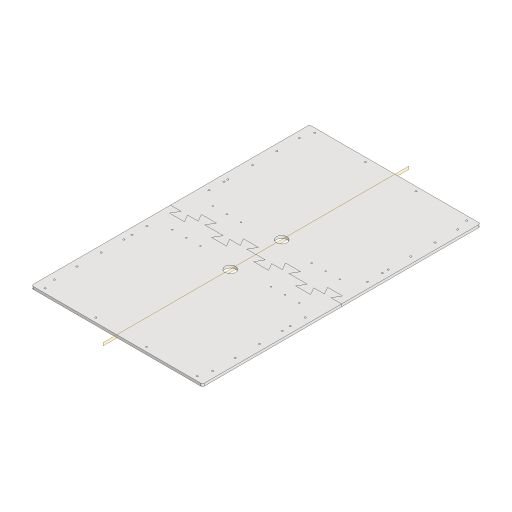
# Autodesk Inventor part: platform
Saved by Autodesk Inventor 2023.2 (Build 272271030, 271C)
## iProperties
Created: 2024-10-30
Part Number: platform
Material: Типовые
Document SubType Name: Modeling
Designer: I9232
Density: 1 g/cm^3
Appearance: По умолчанию
Author: I9232
Autodesk Inventor part; units mm, degrees
ref_plane "XZ Plane" through (0, 0, 0) normal (0, 1, 0) x (-1, 0, 0)
ref_plane "XY Plane" through (0, 0, 0) normal (0, 0, 1) x (1, 0, 0)
sketch "Эскиз1" plane through (0, 0, 0) normal (0, 1, 0) x (-1, 0, 0)
  line L0 (200, 325) -> (-200, 325)
  line L1 (-200, 325) -> (-200, -325)
  line L2 (-200, -325) -> (200, -325)
  line L3 (200, -325) -> (200, 325)
  line L4 (200, 325) -> (-200, -325) construction
  line L5 (-200, 325) -> (200, -325) construction
  point P0 (0, 0)
  dimension "d0" = 650
  dimension "d1" = 400
  constraints: 12 end point, 2 midpoint, 2 parallel, 1 horizontal, 1 perpendicular
  measures "d0" distance of L0.end L1.end
  measures "d1" distance of L1.end L2.end
extrude "Выдавливание1" add sketch "Эскиз1" along normal mid plane 6
fillet "Сопряжение1" radius 4 4 edges at (-200, 0, -325) (200, 0, -325) (200, 0, 325) (-200, 0, 325)
sketch "Эскиз3" plane through (0, 3, 0) normal (0, 1, 0) x (1, 0, 0)
  circle A0 centre (185, -105) radius 2
  arc A1 (-200, -321) -> (-196, -325) centre (-196, -321) ccw projected
  line L0 (-196, -325) -> (196, -325) projected
  arc A2 (196, -325) -> (200, -321) centre (196, -321) ccw projected
  line L1 (200, -321) -> (200, 321) projected
  arc A3 (200, 321) -> (196, 325) centre (196, 321) ccw projected
  line L2 (196, 325) -> (-196, 325) projected
  arc A4 (-196, 325) -> (-200, 321) centre (-196, 321) ccw projected
  line L3 (-200, 321) -> (-200, -321) projected
  line L4 (185, -413) -> (185, 413) construction
  circle A5 centre (-178, 315) radius 2
  line L5 (280, 0) -> (-280, 0) construction
  line L6 (-200, 315) -> (-183.7984, 315) construction
  circle A6 centre (-59.5, 315) radius 2
  circle A7 centre (59, 315) radius 2
  circle A8 centre (177.5, 315) radius 2
  circle A9 centre (185, -286.5) radius 2
  circle A10 centre (185, -233.5) radius 2
  circle A11 centre (185, -177) radius 2
  circle A12 centre (185, -124) radius 2
  circle A13 centre (-178, -315) radius 2
  circle A14 centre (-59.5, -315) radius 2
  circle A15 centre (59, -315) radius 2
  circle A16 centre (177.5, -315) radius 2
  line L7 (0, -50) -> (0, 50) construction
  circle A17 centre (-185, -105) radius 2
  circle A18 centre (-185, -286.5) radius 2
  circle A19 centre (-185, -233.5) radius 2
  circle A20 centre (-185, -177) radius 2
  circle A21 centre (185, 286.5) radius 2
  circle A22 centre (185, 233.5) radius 2
  circle A23 centre (185, 177) radius 2
  circle A24 centre (185, 124) radius 2
  circle A25 centre (-185, 286.5) radius 2
  circle A26 centre (-185, 233.5) radius 2
  circle A27 centre (-185, 177) radius 2
  circle A28 centre (-185, 119) radius 2
  circle A29 centre (185, -70) radius 2
  circle A30 centre (185, 75) radius 2
  circle A31 centre (185, 110) radius 2
  circle A32 centre (-185, -105) radius 2
  circle A33 centre (-185, -70) radius 2
  circle A34 centre (-185, 75) radius 2
  circle A35 centre (-185, 110) radius 2
  circle A36 centre (-185, -124) radius 2
  point P0 (0, 0)
  point P1 (185, 325)
  point P2 (185, -103)
  point P3 (185, -107)
  point P4 (185, -325)
  point P5 (0, 0)
  dimension "d7" = 4
  dimension "d15" = 4
  dimension "d17" = 220
  dimension "d34" = 10
  dimension "d35" = 22
  dimension "d38" = 118.5
  dimension "d43" = 4
  dimension "d44" = 38.5
  dimension "d45" = 4
  dimension "d46" = 4
  dimension "d47" = 4
  dimension "d48" = 53
  dimension "d49" = 53
  dimension "d50" = 56.5
  dimension "d51" = 100
  dimension "d58" = 35
  dimension "d59" = 35
  dimension "d60" = 14
  constraints: 33 centre point, 20 symmetric about line, 6 end point, 3 equal radius, 3 horizontal, 2 midpoint, 2 point on line, 1 vertical, 40 other
  measures "d7" diameter of A0
  measures "d15" diameter of A5
  measures "d17" distance from line of L0 A0.centre
  measures "d34" distance between parallel lines of L2 L6
  measures "d35" distance of L6.start A5.centre
  measures "d38" distance of A5.centre A6.centre
  measures "d43" diameter of A9
  measures "d44" distance from line of L0 A9.centre
  measures "d45" diameter of A10
  measures "d46" diameter of A11
  measures "d47" diameter of A12
  measures "d48" distance of A10.centre A9.centre
  measures "d49" distance of A12.centre A11.centre
  measures "d50" distance of A11.centre A10.centre
  measures "d51" distance of L7.start L7.end
  measures "d58" distance of A29.centre A0.centre
  measures "d59" distance of A31.centre A30.centre
  measures "d60" distance of A24.centre A31.centre
extrude "Выдавливание3" cut sketch "Эскиз3" against normal up to surface (6 mm away) contours A0 | A5 | A6 | A7 | A8 | A9 | A10 | A11 | A12 | A13 | A14 | A15 | A16 | A17 | A18 | A19 | A20 | A21 | A22 | A23 | A24 | A25 | A26 | A27 | A28 | A29 | A30 | A31 | A33 | A34 | A35 | A36
sketch "Эскиз5" plane through (0, -3, 0) normal (0, -1, 0) x (1, 0, 0)
  circle A0 centre (148.4926, 47.4999) radius 1.5999 projected
  circle A1 centre (115.4927, 47.5002) radius 1.6002 projected
  circle A2 centre (82.4926, 47.4999) radius 1.5999 projected
  circle A3 centre (82.4928, -47.4999) radius 1.6002 projected
  circle A4 centre (115.4927, -47.5) radius 1.6001 projected
  circle A5 centre (148.4927, -47.5) radius 1.6001 projected
  circle A6 centre (-82.4927, 47.5) radius 1.5999 projected
  circle A7 centre (-115.4927, 47.5) radius 1.6 projected
  circle A8 centre (-148.4927, 47.4999) radius 1.5999 projected
  circle A9 centre (-148.4927, -47.5) radius 1.6 projected
  circle A10 centre (-115.4927, -47.5) radius 1.5999 projected
  circle A11 centre (-82.4926, -47.5) radius 1.6 projected
  point P0 (0, 0)
extrude "Выдавливание5" cut sketch "Эскиз5" against normal up to surface (6 mm away)
sketch "Эскиз6" plane through (0, -3, 0) normal (0, -1, 0) x (1, 0, 0)
  circle A0 centre (0, 60) radius 12.5
  circle A1 centre (0, -60) radius 12.5
  line L0 (0, 455) -> (0, -455) construction
  point P0 (0, 0)
  dimension "d61" = 25
  dimension "d62" = 25
  dimension "d63" = 60
  dimension "d64" = 60
  constraints: 2 centre point, 2 point on line
  measures "d61" diameter of A0
  measures "d62" diameter of A1
  measures "d63" distance of point (0, 0) A0.centre
  measures "d64" distance of point (0, 0) A1.centre
extrude "Выдавливание6" cut sketch "Эскиз6" against normal up to surface (6 mm away)
sketch "Эскиз7" plane through (0, -3, 0) normal (0, -1, 0) x (1, 0, 0)
  line L0 (200, 321) -> (200, -321) projected
  line L1 (200, 0) -> (175, 0)
  line L2 (175, 0) -> (185, -17.3205)
  line L3 (185, -17.3205) -> (150, -17.3205)
  line L4 (150, -17.3205) -> (160, 0)
  line L5 (160, 0) -> (135, 0)
  line L6 (-200, -321) -> (-200, 321) projected
  line L7 (135, 0) -> (145, 17.3205)
  line L8 (145, 17.3205) -> (110, 17.3205)
  line L9 (110, 17.3205) -> (120, 0)
  line L10 (-280, 0) -> (280, 0) construction
  line L11 (101.6669, 0) -> (76.6669, 0)
  line L12 (76.6669, 0) -> (86.6669, -17.3205)
  line L13 (86.6669, -17.3205) -> (51.6669, -17.3205)
  line L14 (51.6669, -17.3205) -> (61.6669, 0)
  line L15 (61.6669, 0) -> (36.6669, 0)
  line L16 (36.6669, 0) -> (46.6669, 17.3205)
  line L17 (46.6669, 17.3205) -> (11.6669, 17.3205)
  line L18 (11.6669, 17.3205) -> (21.6669, 0)
  line L19 (3.3338, 0) -> (-21.6662, 0)
  line L20 (-21.6662, 0) -> (-11.6662, -17.3205)
  line L21 (-11.6662, -17.3205) -> (-46.6662, -17.3205)
  line L22 (-46.6662, -17.3205) -> (-36.6662, 0)
  line L23 (-36.6662, 0) -> (-61.6662, 0)
  line L24 (-61.6662, 0) -> (-51.6662, 17.3205)
  line L25 (-51.6662, 17.3205) -> (-86.6662, 17.3205)
  line L26 (-86.6662, 17.3205) -> (-76.6662, 0)
  line L27 (-94.9993, 0) -> (-119.9993, 0)
  line L28 (-119.9993, 0) -> (-109.9993, -17.3205)
  line L29 (-109.9993, -17.3205) -> (-144.9993, -17.3205)
  line L30 (-144.9993, -17.3205) -> (-134.9993, 0)
  line L31 (-134.9993, 0) -> (-159.9993, 0)
  line L32 (-159.9993, 0) -> (-149.9993, 17.3205)
  line L33 (-149.9993, 17.3205) -> (-184.9993, 17.3205)
  line L34 (-184.9993, 17.3205) -> (-174.9993, 0)
  line L35 (120, 0) -> (101.6669, 0)
  line L36 (-174.9993, 0) -> (-200, 0)
  line L37 (21.6669, 0) -> (3.3338, 0)
  line L38 (-76.6662, 0) -> (-94.9993, 0)
  point P0 (0, 0)
  dimension "d77" = 15
  dimension "d78" = 25
  dimension "d79" = 15
  dimension "d80" = 60
  dimension "d87" = 60
  dimension "d104" = 60
  dimension "d105" = 60
  dimension "d106" = 15
  dimension "d107" = 35
  dimension "d110" = 98.3331
  constraints: 72 end point, 27 horizontal alignment, 15 collinear, 13 parallel, 4 horizontal, 4 point on line, 2 midpoint, 5 other
  measures "d77" distance of L4.end L1.end
  measures "d78" distance of L1.start L1.end
  measures "d79" distance from line of L0 L2.end
  measures "d80" angle of L2 L1
  measures "d87" angle of L5 L4
  measures "d104" angle to the sketch x axis of L7
  measures "d105" angle to the sketch x axis of L9
  measures "d106" distance of L9.end L5.end
  measures "d107" distance of L7.end L8.end
  measures "d110" distance of L1.start L11.start
split_face "Разделение2"
sketch "Эскиз8" plane through (-196, -3, 325) normal (0, -1, 0) x (1, 0, 0)
  circle A0 centre (381, -75) radius 3.1
  circle A1 centre (381, -45) radius 3.1
  circle A2 centre (381, -15) radius 3.1
  circle A3 centre (351, -15) radius 3.1
  circle A4 centre (11, -15) radius 3.1
  circle A5 centre (41, -15) radius 3.1
  circle A6 centre (11, -45) radius 3.1
  circle A7 centre (11, -75) radius 3.1
  point P0 (196, -325)
  constraints: 8 centre point, 16 other
sketch "Эскиз9" plane through (-196, -3, -325) normal (0, -1, 0) x (1, 0, 0)
  circle A0 centre (381, 15) radius 3.1
  circle A1 centre (351, 15) radius 3.1
  circle A2 centre (381, 45) radius 3.1
  circle A3 centre (381, 75) radius 3.1
  circle A4 centre (41, 15) radius 3.1
  circle A5 centre (11, 15) radius 3.1
  circle A6 centre (11, 45) radius 3.1
  circle A7 centre (11, 75) radius 3.1
  point P0 (196, 325)
  constraints: 8 centre point, 16 other
extrude "Выдавливание7" [suppressed]
extrude "Выдавливание8" [suppressed]
sketch "Эскиз10" plane through (-196, -3, 325) normal (0, -1, 0) x (1, 0, 0)
  circle A0 centre (68.41, -155.97) radius 1.59
  circle A1 centre (116.67, -157.51) radius 1.59
  circle A2 centre (83.61, -105.5) radius 1.55
  circle A3 centre (111.46, -105.5) radius 1.55
  circle A4 centre (68.29, -81.04) radius 1.59
  circle A5 centre (116.67, -74.54) radius 1.59
  circle A6 centre (146.01, -88.2899) radius 1.65
  circle A7 centre (177.0381, -104.4313) radius 1.65
  point P0 (196, -325)
  constraints: 8 centre point, 16 other
extrude "Выдавливание9" [suppressed]
sketch "Эскиз11" plane through (-196, -3, -325) normal (0, -1, 0) x (1, 0, 0)
  circle A0 centre (121, 280) radius 3.15
  circle A1 centre (271, 280) radius 3.15
  circle A2 centre (121, 90) radius 3.15
  circle A3 centre (271, 90) radius 3.15
  point P0 (196, 325)
  constraints: 4 centre point, 8 other
extrude "Выдавливание10" [suppressed]
sketch "Эскиз12" plane through (-196, -3, 325) normal (0, -1, 0) x (1, 0, 0)
  circle A0 centre (255, -10) radius 2
  circle A1 centre (136.5, -10) radius 2
  circle A2 centre (255, -640) radius 2
  circle A3 centre (136.5, -640) radius 2
  point P0 (196, -325)
  constraints: 4 centre point, 8 other
extrude "Выдавливание11" [suppressed]
sketch "Эскиз14" plane through (-196, 3, 325) normal (0, 1, 0) x (1, 0, 0)
  circle A0 centre (11.994, 240.175) radius 2
  line L0 (-4, 325) -> (-4, 4) projected
  line L1 (-4, 325) -> (21.0007, 325) projected
  line L2 (11.994, 325) -> (11.994, 0) construction
  line L3 (21.0007, 325) -> (-4, 325) projected
  line L4 (0, 0) -> (392, 0) projected
  circle A1 centre (11.994, 189.852) radius 2
  point P0 (196, 325)
  dimension "d127" = 15.994
  dimension "d128" = 4
  dimension "d129" = 84.825
  dimension "d130" = 50.323
  constraints: 4 point on line, 2 centre point, 2 end point, 1 equal radius, 1 vertical
  measures "d127" distance between parallel lines of L0 L2
  measures "d128" diameter of A0
  measures "d129" distance from line of L1 A0.centre
  measures "d130" distance of A1.centre A0.centre
extrude "Выдавливание12" [suppressed]
sketch "Эскиз15" plane through (-196, 3, -325) normal (0, 1, 0) x (1, 0, 0)
  line L0 (33.816, 0) -> (33.816, -325) construction
  line L1 (392, 0) -> (0, 0) projected
  line L2 (21.0007, -325) -> (-4, -325) projected
  line L3 (-4, -4) -> (-4, -325) projected
  circle A0 centre (33.816, -78.112) radius 8.462
  circle A1 centre (33.816, -185.601) radius 8.462
  point P0 (196, -325)
  dimension "d133" = 37.816
  dimension "d134" = 16.924
  dimension "d135" = 139.399
  dimension "d136" = 107.489
  constraints: 4 point on line, 2 centre point, 2 end point, 1 equal radius, 1 vertical
  measures "d133" distance between parallel lines of L3 L0
  measures "d134" diameter of A0
  measures "d135" distance from line of L2 A1.centre
  measures "d136" distance of A0.centre A1.centre
extrude "Выдавливание13" [suppressed]
mirror "Зеркальное отражение1" [suppressed]
